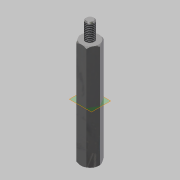
# Autodesk Inventor part: support m3 10
Saved by Autodesk Inventor 2014 (Build 180170000, 170)
## iProperties
Created: 2016-04-01
Part Number: support m3 10
Material: Stainless Steel
Document SubType Name: Modeling
Designer: admin
Density: 8.08 g/cm^3
Appearance: Semi-Polished
Author: admin
Autodesk Inventor part; units mm, degrees
ref_plane "YZ Plane" through (0, 0, 0) normal (1, 0, 0) x (0, 1, 0)
ref_plane "XZ Plane" through (0, 0, 0) normal (0, 1, 0) x (-1, 0, 0)
ref_plane "XY Plane" through (0, 0, 0) normal (0, 0, 1) x (1, 0, 0)
sketch "Sketch1" plane through (0, 0, 0) normal (0, 0, 1) x (1, 0, 0)
  line L0 (1.4434, 2.5) -> (2.8868, 0)
  line L1 (2.8868, 0) -> (1.4434, -2.5)
  line L2 (1.4434, -2.5) -> (-1.4434, -2.5)
  line L3 (-1.4434, -2.5) -> (-2.8868, 0)
  line L4 (-2.8868, 0) -> (-1.4434, 2.5)
  line L5 (-1.4434, 2.5) -> (1.4434, 2.5)
  point P0 (0, 0)
  point P1 (0, 0)
  dimension "d0" = 5
  constraints: 12 end point, 1 coincident, 13 other
  measures "d0" distance between parallel lines of L2 L5
extrude "Extrusion1" add sketch "Sketch1" along normal blind 30
sketch "Sketch3" plane through (0, 0, 0) normal (0, 0, -1) x (-1, 0, 0)
  line L0 (1.4434, 2.5) -> (-1.4434, 2.5) projected
  circle A0 centre (0, 0) radius 2.5
  constraints: 1 centre point, 1 coincident, 1 tangent
hole "Hole1" at (0, 0, 0) direction (0, 0, 1) diameter 2.459 end through all thread size "M3x0.5" class "6H" standard "ISO Metric profile"
chamfer "Chamfer2" distance 0.5 angle 45 1 edges at (0, -1.2295, 0)
sketch "Sketch4" plane through (0, 0, 0) normal (0, 0, -1) x (-1, 0, 0)
  circle A0 centre (0, 0) radius 1.7295 projected
  circle A1 centre (0, 0) radius 2.5
  circle A2 centre (0, 0) radius 6
  constraints: 2 centre point, 2 coincident
extrude "Extrusion3" cut sketch "Sketch4" against normal blind 1 draft -45 contours A2
ref_plane "Work Plane1" through (0, 0, 15) normal (0, 0, -1) x (-1, 0, 0)
mirror "Mirror2" about plane through (0, 0, 15) normal (0, 0, -1) of "Extrusion3"
sketch "Sketch5" plane through (0, 0, 30) normal (0, 0, 1) x (1, 0, 0)
  circle A0 centre (0, 0) radius 1.2295 projected
extrude "Extrusion4" add sketch "Sketch5" along normal blind 5 and the other way blind 25
thread "Thread2" size "M2.5x0.45" class "6g" standard "ANSI Metric M Profile" full length
chamfer "Chamfer4" distance 0.3 angle 45 1 edges at (-1.2295, 0, 35)
body "Solid1"
